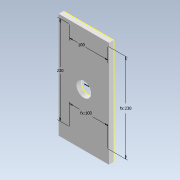
# Autodesk Inventor part: placa superior
Saved by Autodesk Inventor 2021 (Build 250183000, 183)
## iProperties
Created: 2021-08-20
Part Number: placa superior
Material: Generic
Document SubType Name: Modeling
Designer: Andrés Holguín
Density: 1 g/cm^3
Appearance: Default
Author: Andrés Holguín
Autodesk Inventor part; units mm, degrees
ref_plane "YZ Plane" through (0, 0, 0) normal (1, 0, 0) x (0, 1, 0)
ref_plane "XZ Plane" through (0, 0, 0) normal (0, 1, 0) x (-1, 0, 0)
ref_plane "XY Plane" through (0, 0, 0) normal (0, 0, 1) x (1, 0, 0)
sketch "Sketch1" plane through (0, 0, 0) normal (0, 0, 1) x (1, 0, 0)
  line L0 (-67.4611, 97.9784) -> (62.5389, 97.9784)
  line L1 (62.5389, 97.9784) -> (62.5389, -175.0216)
  line L2 (62.5389, -175.0216) -> (-67.4611, -175.0216)
  line L3 (-67.4611, -175.0216) -> (-67.4611, 97.9784)
  circle A0 centre (-2.4611, -38.5216) radius 19.05
  line L4 (-67.4611, -38.5216) -> (62.5389, -38.5216) construction
  line L5 (-2.4611, 97.9784) -> (-2.4611, -175.0216) construction
  point P0 (0, 0)
  point P1 (-2.4611, -38.5216)
  dimension "d0" = 38.1
  dimension "d3" = 130
  dimension "d4" = 273
  constraints: 12 end point, 5 midpoint, 2 parallel, 1 centre point, 1 coincident, 1 horizontal, 1 perpendicular
  measures "d0" diameter of A0
  measures "d3" distance of L0.start L0.end
  measures "d4" distance of L2.end L0.start
extrude "Extrusion1" add sketch "Sketch1" along normal blind 12.7
sketch "Sketch2" plane through (0, 0, 0) normal (0, 0, -1) x (-1, 0, 0)
  line L0 (67.4611, -175.0216) -> (-62.5389, -175.0216) projected
  line L1 (67.4611, 97.9784) -> (67.4611, -175.0216) projected
  line L2 (-62.5389, 97.9784) -> (67.4611, 97.9784) projected
  line L3 (-62.5389, -175.0216) -> (-62.5389, 97.9784) projected
  circle A0 centre (2.4611, -38.5216) radius 19.05 projected
  line L4 (2.4611, -38.5216) -> (2.4611, -25.0418)
  line L5 (2.4611, -25.0418) -> (2.4611, -38.5216)
  line L6 (14.6161, -38.5216) -> (2.4611, -38.5216)
  point P0 (0, 0)
  point P1 (42.4611, 76.4784)
  point P2 (-37.5389, 76.4784)
  point P3 (-37.5389, -153.5216)
  point P4 (42.4611, -153.5216)
  dimension "d5" = 230
  dimension "d6" = 80
  dimension "d7" = 80
  dimension "d8" = 230
  constraints: 6 end point, 2 symmetric about line, 1 collinear, 1 perpendicular, 1 vertical
  measures "d5" distance of point (42.461, -153.522) point (42.461, 76.478)
  measures "d6" distance of point (42.461, 76.478) point (-37.539, 76.478)
  measures "d7" distance of point (42.461, -153.522) point (-37.539, -153.522)
  measures "d8" distance of point (-37.539, 76.478) point (-37.539, -153.522)
hole "Hole1" at (-42.4611, 76.4784, 0) at (37.5389, 76.4784, 0) at (37.5389, -153.5216, 0) at (-42.4611, -153.5216, 0) direction (0, 0, 1) diameter 12 end through all
equation "\"d7\" = d6"
equation "\"d8\" = d5"
body "Solid1"
